Autodesk Fusion 360 part; units mm, degrees
(part 2 of 2)
sketch "Sketch5" plane through (0, 0, 0) normal (0, 1, 0) x (1, 0, 0)
  line L0 (-114.6631, -42.9541) -> (-114.6631, -45.4541)
  line L1 (-114.6631, -45.4541) -> (-84.6631, -45.4541)
  line L2 (-84.6631, -45.4541) -> (-84.6631, -42.9541)
  line L3 (-84.6631, -42.9541) -> (-114.6631, -42.9541)
  line L4 (-181.3297, -42.9541) -> (-181.3297, -45.4541)
  line L5 (-181.3297, -45.4541) -> (-151.3297, -45.4541)
  line L6 (-151.3297, -45.4541) -> (-151.3297, -42.9541)
  line L7 (-151.3297, -42.9541) -> (-181.3297, -42.9541)
  line L8 (-247.9964, -42.9541) -> (-247.9964, -45.4541)
  line L9 (-247.9964, -45.4541) -> (-217.9964, -45.4541)
  line L10 (-217.9964, -45.4541) -> (-217.9964, -42.9541)
  line L11 (-217.9964, -42.9541) -> (-247.9964, -42.9541)
  line L12 (-314.6631, -42.9541) -> (-314.6631, -45.4541)
  line L13 (-314.6631, -45.4541) -> (-284.6631, -45.4541)
  line L14 (-284.6631, -45.4541) -> (-284.6631, -42.9541)
  line L15 (-284.6631, -42.9541) -> (-314.6631, -42.9541)
  line L16 (-181.3297, -80.9541) -> (-181.3297, -83.4541)
  line L17 (-181.3297, -83.4541) -> (-151.3297, -83.4541)
  line L18 (-151.3297, -83.4541) -> (-151.3297, -80.9541)
  line L19 (-151.3297, -80.9541) -> (-181.3297, -80.9541)
  line L20 (-114.6631, -80.9541) -> (-114.6631, -83.4541)
  line L21 (-114.6631, -83.4541) -> (-84.6631, -83.4541)
  line L22 (-84.6631, -83.4541) -> (-84.6631, -80.9541)
  line L23 (-84.6631, -80.9541) -> (-114.6631, -80.9541)
  line L24 (-314.6631, -156.9541) -> (-314.6631, -159.4541)
  line L25 (-314.6631, -159.4541) -> (-284.6631, -159.4541)
  line L26 (-284.6631, -159.4541) -> (-284.6631, -156.9541)
  line L27 (-284.6631, -156.9541) -> (-314.6631, -156.9541)
  line L28 (-114.6631, -194.9541) -> (-114.6631, -197.4541)
  line L29 (-114.6631, -197.4541) -> (-84.6631, -197.4541)
  line L30 (-84.6631, -197.4541) -> (-84.6631, -194.9541)
  line L31 (-84.6631, -194.9541) -> (-114.6631, -194.9541)
  line L32 (-181.3297, -194.9541) -> (-181.3297, -197.4541)
  line L33 (-181.3297, -197.4541) -> (-151.3297, -197.4541)
  line L34 (-151.3297, -197.4541) -> (-151.3297, -194.9541)
  line L35 (-151.3297, -194.9541) -> (-181.3297, -194.9541)
  line L36 (-247.9964, -194.9541) -> (-247.9964, -197.4541)
  line L37 (-247.9964, -197.4541) -> (-217.9964, -197.4541)
  line L38 (-217.9964, -197.4541) -> (-217.9964, -194.9541)
  line L39 (-217.9964, -194.9541) -> (-247.9964, -194.9541)
  line L40 (-314.6631, -194.9541) -> (-314.6631, -197.4541)
  line L41 (-314.6631, -197.4541) -> (-284.6631, -197.4541)
  line L42 (-284.6631, -197.4541) -> (-284.6631, -194.9541)
  line L43 (-284.6631, -194.9541) -> (-314.6631, -194.9541)
  line L44 (-114.6631, -232.9541) -> (-114.6631, -235.4541)
  line L45 (-114.6631, -235.4541) -> (-84.6631, -235.4541)
  line L46 (-84.6631, -235.4541) -> (-84.6631, -232.9541)
  line L47 (-84.6631, -232.9541) -> (-114.6631, -232.9541)
  line L48 (-181.3297, -232.9541) -> (-181.3297, -235.4541)
  line L49 (-181.3297, -235.4541) -> (-151.3297, -235.4541)
  line L50 (-151.3297, -235.4541) -> (-151.3297, -232.9541)
  line L51 (-151.3297, -232.9541) -> (-181.3297, -232.9541)
  line L52 (-247.9964, -232.9541) -> (-247.9964, -235.4541)
  line L53 (-247.9964, -235.4541) -> (-217.9964, -235.4541)
  line L54 (-217.9964, -235.4541) -> (-217.9964, -232.9541)
  line L55 (-217.9964, -232.9541) -> (-247.9964, -232.9541)
  line L56 (-314.6631, -232.9541) -> (-314.6631, -235.4541)
  line L57 (-314.6631, -235.4541) -> (-284.6631, -235.4541)
  line L58 (-284.6631, -235.4541) -> (-284.6631, -232.9541)
  line L59 (-284.6631, -232.9541) -> (-314.6631, -232.9541)
  line L60 (-314.6631, -80.9541) -> (-314.6631, -83.4541)
  line L61 (-314.6631, -83.4541) -> (-284.6631, -83.4541)
  line L62 (-284.6631, -83.4541) -> (-284.6631, -80.9541)
  line L63 (-284.6631, -80.9541) -> (-314.6631, -80.9541)
  line L64 (-247.9964, -118.9541) -> (-247.9964, -121.4541)
  line L65 (-247.9964, -121.4541) -> (-217.9964, -121.4541)
  line L66 (-217.9964, -121.4541) -> (-217.9964, -118.9541)
  line L67 (-217.9964, -118.9541) -> (-247.9964, -118.9541)
  line L68 (-247.9964, -80.9541) -> (-247.9964, -83.4541)
  line L69 (-247.9964, -83.4541) -> (-217.9964, -83.4541)
  line L70 (-217.9964, -83.4541) -> (-217.9964, -80.9541)
  line L71 (-217.9964, -80.9541) -> (-247.9964, -80.9541)
  line L72 (-181.3297, -118.9541) -> (-181.3297, -121.4541)
  line L73 (-181.3297, -121.4541) -> (-151.3297, -121.4541)
  line L74 (-151.3297, -121.4541) -> (-151.3297, -118.9541)
  line L75 (-151.3297, -118.9541) -> (-181.3297, -118.9541)
  line L76 (-114.6631, -118.9541) -> (-114.6631, -121.4541)
  line L77 (-114.6631, -121.4541) -> (-84.6631, -121.4541)
  line L78 (-84.6631, -121.4541) -> (-84.6631, -118.9541)
  line L79 (-84.6631, -118.9541) -> (-114.6631, -118.9541)
  line L80 (-247.9964, -156.9541) -> (-247.9964, -159.4541)
  line L81 (-247.9964, -159.4541) -> (-217.9964, -159.4541)
  line L82 (-217.9964, -159.4541) -> (-217.9964, -156.9541)
  line L83 (-217.9964, -156.9541) -> (-247.9964, -156.9541)
  line L84 (-181.3297, -156.9541) -> (-181.3297, -159.4541)
  line L85 (-181.3297, -159.4541) -> (-151.3297, -159.4541)
  line L86 (-151.3297, -159.4541) -> (-151.3297, -156.9541)
  line L87 (-151.3297, -156.9541) -> (-181.3297, -156.9541)
  line L88 (-114.6631, -156.9541) -> (-114.6631, -159.4541)
  line L89 (-114.6631, -159.4541) -> (-84.6631, -159.4541)
  line L90 (-84.6631, -159.4541) -> (-84.6631, -156.9541)
  line L91 (-84.6631, -156.9541) -> (-114.6631, -156.9541)
  line L92 (-314.6631, -118.9541) -> (-314.6631, -121.4541)
  line L93 (-314.6631, -121.4541) -> (-284.6631, -121.4541)
  line L94 (-284.6631, -121.4541) -> (-284.6631, -118.9541)
  line L95 (-284.6631, -118.9541) -> (-314.6631, -118.9541)
  line L96 (-347.5, -182.5558) -> (-350, -182.5558)
  line L97 (-350, -182.5558) -> (-350, -154.875)
  line L98 (-350, -154.875) -> (-347.5, -154.875)
  line L99 (-347.5, -154.875) -> (-347.5, -115.125)
  line L100 (-347.5, -115.125) -> (-350, -115.125)
  line L101 (-350, -115.125) -> (-350, -87.4442)
  line L102 (-350, -87.4442) -> (-347.5, -87.4442)
  line L103 (-347.5, -87.4442) -> (-347.5, -47.6942)
  line L104 (-347.5, -47.6942) -> (-350, -47.6942)
  line L105 (-350, -47.6942) -> (-350, -10)
  line L106 (-350, -10) -> (-316.8881, -10)
  line L107 (-316.8881, -10) -> (-316.8881, -12.5)
  line L108 (-316.8881, -12.5) -> (-277.1381, -12.5)
  line L109 (-277.1381, -12.5) -> (-277.1381, -10)
  line L110 (-277.1381, -10) -> (-219.9429, -10)
  line L111 (-219.9429, -10) -> (-219.9429, -12.5)
  line L112 (-219.9429, -12.5) -> (-180.1929, -12.5)
  line L113 (-180.1929, -12.5) -> (-180.1929, -10)
  line L114 (-180.1929, -10) -> (-122.8387, -10)
  line L115 (-122.8387, -10) -> (-122.8387, -12.5)
  line L116 (-122.8387, -12.5) -> (-83.0887, -12.5)
  line L117 (-83.0887, -12.5) -> (-83.0887, -10)
  line L118 (-83.0887, -10) -> (-50, -10)
  line L119 (-50, -10) -> (-50, -47.6942)
  line L120 (-50, -47.6942) -> (-52.5, -47.6942)
  line L121 (-52.5, -47.6942) -> (-52.5, -87.4442)
  line L122 (-52.5, -87.4442) -> (-50, -87.4442)
  line L123 (-50, -87.4442) -> (-50, -115.125)
  line L124 (-50, -115.125) -> (-52.5, -115.125)
  line L125 (-52.5, -115.125) -> (-52.5, -154.875)
  line L126 (-52.5, -154.875) -> (-50, -154.875)
  line L127 (-50, -154.875) -> (-50, -182.5558)
  line L128 (-50, -182.5558) -> (-52.5, -182.5558)
  line L129 (-52.5, -182.5558) -> (-52.5, -222.3058)
  line L130 (-52.5, -222.3058) -> (-50, -222.3058)
  line L131 (-50, -222.3058) -> (-50, -260)
  line L132 (-50, -260) -> (-350, -260)
  line L133 (-350, -260) -> (-350, -222.3058)
  line L134 (-350, -222.3058) -> (-347.5, -222.3058)
  line L135 (-347.5, -222.3058) -> (-347.5, -182.5558)
  line L136 (-350, -382.5617) -> (-350, -362.5617)
  line L137 (-350, -362.5617) -> (-314.6631, -362.5617)
  line L138 (-314.6631, -362.5617) -> (-314.6631, -282.5617)
  line L139 (-314.6631, -282.5617) -> (-284.6631, -282.5617)
  line L140 (-284.6631, -282.5617) -> (-284.6631, -362.5617)
  line L141 (-284.6631, -362.5617) -> (-247.9964, -362.5617)
  line L142 (-247.9964, -362.5617) -> (-247.9964, -282.5617)
  line L143 (-247.9964, -282.5617) -> (-217.9964, -282.5617)
  line L144 (-217.9964, -282.5617) -> (-217.9964, -362.5617)
  line L145 (-217.9964, -362.5617) -> (-181.3297, -362.5617)
  line L146 (-181.3297, -362.5617) -> (-181.3297, -282.5617)
  line L147 (-181.3297, -282.5617) -> (-151.3297, -282.5617)
  line L148 (-151.3297, -282.5617) -> (-151.3297, -362.5617)
  line L149 (-151.3297, -362.5617) -> (-114.6631, -362.5617)
  line L150 (-114.6631, -362.5617) -> (-114.6631, -282.5617)
  line L151 (-114.6631, -282.5617) -> (-84.6631, -282.5617)
  line L152 (-84.6631, -282.5617) -> (-84.6631, -362.5617)
  line L153 (-84.6631, -362.5617) -> (-50, -362.5617)
  line L154 (-50, -362.5617) -> (-50, -382.5617)
  arc A0 (-60, -392.5617) -> (-50, -382.5617) centre (-60, -382.5617) ccw
  line L155 (-60, -392.5617) -> (-340, -392.5617)
  arc A1 (-350, -382.5617) -> (-340, -392.5617) centre (-340, -382.5617) ccw
  line L156 (0, -357.5617) -> (0, -337.5617)
  line L157 (0, -337.5617) -> (35.3369, -337.5617)
  line L158 (35.3369, -337.5617) -> (35.3369, -257.5617)
  line L159 (35.3369, -257.5617) -> (65.3369, -257.5617)
  line L160 (65.3369, -257.5617) -> (65.3369, -337.5617)
  line L161 (65.3369, -337.5617) -> (102.0036, -337.5617)
  line L162 (102.0036, -337.5617) -> (102.0036, -257.5617)
  line L163 (102.0036, -257.5617) -> (132.0036, -257.5617)
  line L164 (132.0036, -257.5617) -> (132.0036, -337.5617)
  line L165 (132.0036, -337.5617) -> (168.6703, -337.5617)
  line L166 (168.6703, -337.5617) -> (168.6703, -257.5617)
  line L167 (168.6703, -257.5617) -> (198.6703, -257.5617)
  line L168 (198.6703, -257.5617) -> (198.6703, -337.5617)
  line L169 (198.6703, -337.5617) -> (235.3369, -337.5617)
  line L170 (235.3369, -337.5617) -> (235.3369, -257.5617)
  line L171 (235.3369, -257.5617) -> (265.3369, -257.5617)
  line L172 (265.3369, -257.5617) -> (265.3369, -337.5617)
  line L173 (265.3369, -337.5617) -> (300, -337.5617)
  line L174 (300, -337.5617) -> (300, -357.5617)
  arc A2 (290, -367.5617) -> (300, -357.5617) centre (290, -357.5617) ccw
  line L175 (290, -367.5617) -> (10, -367.5617)
  arc A3 (0, -357.5617) -> (10, -367.5617) centre (10, -357.5617) ccw
  line L176 (235.3369, -32.9541) -> (235.3369, -35.4541)
  line L177 (235.3369, -35.4541) -> (265.3369, -35.4541)
  line L178 (265.3369, -35.4541) -> (265.3369, -32.9541)
  line L179 (265.3369, -32.9541) -> (235.3369, -32.9541)
  line L180 (168.6703, -32.9541) -> (168.6703, -35.4541)
  line L181 (168.6703, -35.4541) -> (198.6703, -35.4541)
  line L182 (198.6703, -35.4541) -> (198.6703, -32.9541)
  line L183 (198.6703, -32.9541) -> (168.6703, -32.9541)
  line L184 (102.0036, -32.9541) -> (102.0036, -35.4541)
  line L185 (102.0036, -35.4541) -> (132.0036, -35.4541)
  line L186 (132.0036, -35.4541) -> (132.0036, -32.9541)
  line L187 (132.0036, -32.9541) -> (102.0036, -32.9541)
  line L188 (35.3369, -32.9541) -> (35.3369, -35.4541)
  line L189 (35.3369, -35.4541) -> (65.3369, -35.4541)
  line L190 (65.3369, -35.4541) -> (65.3369, -32.9541)
  line L191 (65.3369, -32.9541) -> (35.3369, -32.9541)
  line L192 (168.6703, -70.9541) -> (168.6703, -73.4541)
  line L193 (168.6703, -73.4541) -> (198.6703, -73.4541)
  line L194 (198.6703, -73.4541) -> (198.6703, -70.9541)
  line L195 (198.6703, -70.9541) -> (168.6703, -70.9541)
  line L196 (235.3369, -70.9541) -> (235.3369, -73.4541)
  line L197 (235.3369, -73.4541) -> (265.3369, -73.4541)
  line L198 (265.3369, -73.4541) -> (265.3369, -70.9541)
  line L199 (265.3369, -70.9541) -> (235.3369, -70.9541)
  line L200 (35.3369, -146.9541) -> (35.3369, -149.4541)
  line L201 (35.3369, -149.4541) -> (65.3369, -149.4541)
  line L202 (65.3369, -149.4541) -> (65.3369, -146.9541)
  line L203 (65.3369, -146.9541) -> (35.3369, -146.9541)
  line L204 (235.3369, -184.9541) -> (235.3369, -187.4541)
  line L205 (235.3369, -187.4541) -> (265.3369, -187.4541)
  line L206 (265.3369, -187.4541) -> (265.3369, -184.9541)
  line L207 (265.3369, -184.9541) -> (235.3369, -184.9541)
  line L208 (168.6703, -184.9541) -> (168.6703, -187.4541)
  line L209 (168.6703, -187.4541) -> (198.6703, -187.4541)
  line L210 (198.6703, -187.4541) -> (198.6703, -184.9541)
  line L211 (198.6703, -184.9541) -> (168.6703, -184.9541)
  line L212 (102.0036, -184.9541) -> (102.0036, -187.4541)
  line L213 (102.0036, -187.4541) -> (132.0036, -187.4541)
  line L214 (132.0036, -187.4541) -> (132.0036, -184.9541)
  line L215 (132.0036, -184.9541) -> (102.0036, -184.9541)
  line L216 (35.3369, -184.9541) -> (35.3369, -187.4541)
  line L217 (35.3369, -187.4541) -> (65.3369, -187.4541)
  line L218 (65.3369, -187.4541) -> (65.3369, -184.9541)
  line L219 (65.3369, -184.9541) -> (35.3369, -184.9541)
  line L220 (235.3369, -222.9541) -> (235.3369, -225.4541)
  line L221 (235.3369, -225.4541) -> (265.3369, -225.4541)
  line L222 (265.3369, -225.4541) -> (265.3369, -222.9541)
  line L223 (265.3369, -222.9541) -> (235.3369, -222.9541)
  line L224 (168.6703, -222.9541) -> (168.6703, -225.4541)
  line L225 (168.6703, -225.4541) -> (198.6703, -225.4541)
  line L226 (198.6703, -225.4541) -> (198.6703, -222.9541)
  line L227 (198.6703, -222.9541) -> (168.6703, -222.9541)
  line L228 (102.0036, -222.9541) -> (102.0036, -225.4541)
  line L229 (102.0036, -225.4541) -> (132.0036, -225.4541)
  line L230 (132.0036, -225.4541) -> (132.0036, -222.9541)
  line L231 (132.0036, -222.9541) -> (102.0036, -222.9541)
  line L232 (35.3369, -222.9541) -> (35.3369, -225.4541)
  line L233 (35.3369, -225.4541) -> (65.3369, -225.4541)
  line L234 (65.3369, -225.4541) -> (65.3369, -222.9541)
  line L235 (65.3369, -222.9541) -> (35.3369, -222.9541)
  line L236 (35.3369, -70.9541) -> (35.3369, -73.4541)
  line L237 (35.3369, -73.4541) -> (65.3369, -73.4541)
  line L238 (65.3369, -73.4541) -> (65.3369, -70.9541)
  line L239 (65.3369, -70.9541) -> (35.3369, -70.9541)
  line L240 (102.0036, -108.9541) -> (102.0036, -111.4541)
  line L241 (102.0036, -111.4541) -> (132.0036, -111.4541)
  line L242 (132.0036, -111.4541) -> (132.0036, -108.9541)
  line L243 (132.0036, -108.9541) -> (102.0036, -108.9541)
  line L244 (102.0036, -70.9541) -> (102.0036, -73.4541)
  line L245 (102.0036, -73.4541) -> (132.0036, -73.4541)
  line L246 (132.0036, -73.4541) -> (132.0036, -70.9541)
  line L247 (132.0036, -70.9541) -> (102.0036, -70.9541)
  line L248 (168.6703, -108.9541) -> (168.6703, -111.4541)
  line L249 (168.6703, -111.4541) -> (198.6703, -111.4541)
  line L250 (198.6703, -111.4541) -> (198.6703, -108.9541)
  line L251 (198.6703, -108.9541) -> (168.6703, -108.9541)
  line L252 (235.3369, -108.9541) -> (235.3369, -111.4541)
  line L253 (235.3369, -111.4541) -> (265.3369, -111.4541)
  line L254 (265.3369, -111.4541) -> (265.3369, -108.9541)
  line L255 (265.3369, -108.9541) -> (235.3369, -108.9541)
  line L256 (102.0036, -146.9541) -> (102.0036, -149.4541)
  line L257 (102.0036, -149.4541) -> (132.0036, -149.4541)
  line L258 (132.0036, -149.4541) -> (132.0036, -146.9541)
  line L259 (132.0036, -146.9541) -> (102.0036, -146.9541)
  line L260 (168.6703, -146.9541) -> (168.6703, -149.4541)
  line L261 (168.6703, -149.4541) -> (198.6703, -149.4541)
  line L262 (198.6703, -149.4541) -> (198.6703, -146.9541)
  line L263 (198.6703, -146.9541) -> (168.6703, -146.9541)
  line L264 (235.3369, -146.9541) -> (235.3369, -149.4541)
  line L265 (235.3369, -149.4541) -> (265.3369, -149.4541)
  line L266 (265.3369, -149.4541) -> (265.3369, -146.9541)
  line L267 (265.3369, -146.9541) -> (235.3369, -146.9541)
  line L268 (35.3369, -108.9541) -> (35.3369, -111.4541)
  line L269 (35.3369, -111.4541) -> (65.3369, -111.4541)
  line L270 (65.3369, -111.4541) -> (65.3369, -108.9541)
  line L271 (65.3369, -108.9541) -> (35.3369, -108.9541)
  line L272 (2.5, -172.5558) -> (0, -172.5558)
  line L273 (0, -172.5558) -> (0, -144.875)
  line L274 (0, -144.875) -> (2.5, -144.875)
  line L275 (2.5, -144.875) -> (2.5, -105.125)
  line L276 (2.5, -105.125) -> (0, -105.125)
  line L277 (0, -105.125) -> (0, -77.4442)
  line L278 (0, -77.4442) -> (2.5, -77.4442)
  line L279 (2.5, -77.4442) -> (2.5, -37.6942)
  line L280 (2.5, -37.6942) -> (0, -37.6942)
  line L281 (0, -37.6942) -> (0, 0)
  line L282 (0, 0) -> (33.1119, 0)
  line L283 (33.1119, 0) -> (33.1119, -2.5)
  line L284 (33.1119, -2.5) -> (72.8619, -2.5)
  line L285 (72.8619, -2.5) -> (72.8619, 0)
  line L286 (72.8619, 0) -> (130.0571, 0)
  line L287 (130.0571, 0) -> (130.0571, -2.5)
  line L288 (130.0571, -2.5) -> (169.8071, -2.5)
  line L289 (169.8071, -2.5) -> (169.8071, 0)
  line L290 (169.8071, 0) -> (227.1613, 0)
  line L291 (227.1613, 0) -> (227.1613, -2.5)
  line L292 (227.1613, -2.5) -> (266.9113, -2.5)
  line L293 (266.9113, -2.5) -> (266.9113, 0)
  line L294 (266.9113, 0) -> (300, 0)
  line L295 (300, 0) -> (300, -37.6942)
  line L296 (300, -37.6942) -> (297.5, -37.6942)
  line L297 (297.5, -37.6942) -> (297.5, -77.4442)
  line L298 (297.5, -77.4442) -> (300, -77.4442)
  line L299 (300, -77.4442) -> (300, -105.125)
  line L300 (300, -105.125) -> (297.5, -105.125)
  line L301 (297.5, -105.125) -> (297.5, -144.875)
  line L302 (297.5, -144.875) -> (300, -144.875)
  line L303 (300, -144.875) -> (300, -172.5558)
  line L304 (300, -172.5558) -> (297.5, -172.5558)
  line L305 (297.5, -172.5558) -> (297.5, -212.3058)
  line L306 (297.5, -212.3058) -> (300, -212.3058)
  line L307 (300, -212.3058) -> (300, -250)
  line L308 (300, -250) -> (0, -250)
  line L309 (0, -250) -> (0, -212.3058)
  line L310 (0, -212.3058) -> (2.5, -212.3058)
  line L311 (2.5, -212.3058) -> (2.5, -172.5558)
  line L312 (296.4708, 56.207) -> (296.4708, 12.1817)
  line L313 (296.4708, 12.1817) -> (265.8821, 12.1817)
  line L314 (265.8821, 12.1817) -> (265.8821, 9.6817)
  line L315 (265.8821, 9.6817) -> (225.8821, 9.6817)
  line L316 (225.8821, 9.6817) -> (225.8821, 12.1817)
  line L317 (225.8821, 12.1817) -> (168.5279, 12.1817)
  line L318 (168.5279, 12.1817) -> (168.5279, 9.6817)
  line L319 (168.5279, 9.6817) -> (129.2779, 9.6817)
  line L320 (129.2779, 9.6817) -> (129.2779, 12.1817)
  line L321 (129.2779, 12.1817) -> (72.0827, 12.1817)
  line L322 (72.0827, 12.1817) -> (72.0827, 9.6817)
  line L323 (72.0827, 9.6817) -> (32.0827, 9.6817)
  line L324 (32.0827, 9.6817) -> (32.0827, 12.1817)
  line L325 (32.0827, 12.1817) -> (1.4708, 12.1817)
  line L326 (1.4708, 12.1817) -> (1.4708, 56.207)
  line L327 (1.4708, 56.207) -> (-1.0292, 56.207)
  line L328 (-1.0292, 56.207) -> (-1.0292, 96.207)
  line L329 (-1.0292, 96.207) -> (1.4708, 96.207)
  line L330 (1.4708, 96.207) -> (1.4708, 139.6817)
  line L331 (1.4708, 139.6817) -> (-1.0292, 139.6817)
  line L332 (-1.0292, 139.6817) -> (-1.0292, 179.6817)
  line L333 (-1.0292, 179.6817) -> (1.4708, 179.6817)
  line L334 (1.4708, 179.6817) -> (1.4708, 223.1564)
  line L335 (1.4708, 223.1564) -> (-1.0292, 223.1564)
  line L336 (-1.0292, 223.1564) -> (-1.0292, 263.1564)
  line L337 (-1.0292, 263.1564) -> (1.4708, 263.1564)
  line L338 (1.4708, 263.1564) -> (1.4708, 307.1817)
  line L339 (1.4708, 307.1817) -> (32.0827, 307.1817)
  line L340 (32.0827, 307.1817) -> (32.0827, 309.6817)
  line L341 (32.0827, 309.6817) -> (72.0827, 309.6817)
  line L342 (72.0827, 309.6817) -> (72.0827, 307.1817)
  line L343 (72.0827, 307.1817) -> (129.2779, 307.1817)
  line L344 (129.2779, 307.1817) -> (129.2779, 309.6817)
  line L345 (129.2779, 309.6817) -> (168.5279, 309.6817)
  line L346 (168.5279, 309.6817) -> (168.5279, 307.1817)
  line L347 (168.5279, 307.1817) -> (225.8821, 307.1817)
  line L348 (225.8821, 307.1817) -> (225.8821, 309.6817)
  line L349 (225.8821, 309.6817) -> (265.8821, 309.6817)
  line L350 (265.8821, 309.6817) -> (265.8821, 307.1817)
  line L351 (265.8821, 307.1817) -> (296.4708, 307.1817)
  line L352 (296.4708, 307.1817) -> (296.4708, 263.1564)
  line L353 (296.4708, 263.1564) -> (298.9708, 263.1564)
  line L354 (298.9708, 263.1564) -> (298.9708, 223.1564)
  line L355 (298.9708, 223.1564) -> (296.4708, 223.1564)
  line L356 (296.4708, 223.1564) -> (296.4708, 179.6817)
  line L357 (296.4708, 179.6817) -> (298.9708, 179.6817)
  line L358 (298.9708, 179.6817) -> (298.9708, 139.6817)
  line L359 (298.9708, 139.6817) -> (296.4708, 139.6817)
  line L360 (296.4708, 139.6817) -> (296.4708, 96.207)
  line L361 (296.4708, 96.207) -> (298.9708, 96.207)
  line L362 (298.9708, 96.207) -> (298.9708, 56.207)
  line L363 (298.9708, 56.207) -> (296.4708, 56.207)
  line L364 (-18.915, 96.082) -> (-21.415, 96.082)
  line L365 (-21.415, 96.082) -> (-21.415, 56.332)
  line L366 (-21.415, 56.332) -> (-18.915, 56.332)
  line L367 (-18.915, 56.332) -> (-18.915, 12.1817)
  line L368 (-18.915, 12.1817) -> (-56.6092, 12.1817)
  line L369 (-56.6092, 12.1817) -> (-56.6092, 9.6817)
  line L370 (-56.6092, 9.6817) -> (-96.6092, 9.6817)
  line L371 (-96.6092, 9.6817) -> (-96.6092, 12.1817)
  line L372 (-96.6092, 12.1817) -> (-123.54, 12.1817)
  line L373 (-123.54, 12.1817) -> (-123.54, 9.6817)
  line L374 (-123.54, 9.6817) -> (-163.54, 9.6817)
  line L375 (-163.54, 9.6817) -> (-163.54, 12.1817)
  line L376 (-163.54, 12.1817) -> (-191.2208, 12.1817)
  line L377 (-191.2208, 12.1817) -> (-191.2208, 9.6817)
  line L378 (-191.2208, 9.6817) -> (-231.2208, 9.6817)
  line L379 (-231.2208, 9.6817) -> (-231.2208, 12.1817)
  line L380 (-231.2208, 12.1817) -> (-268.915, 12.1817)
  line L381 (-268.915, 12.1817) -> (-268.915, 307.1817)
  line L382 (-268.915, 307.1817) -> (-231.2208, 307.1817)
  line L383 (-231.2208, 307.1817) -> (-231.2208, 309.6817)
  line L384 (-231.2208, 309.6817) -> (-191.2208, 309.6817)
  line L385 (-191.2208, 309.6817) -> (-191.2208, 307.1817)
  line L386 (-191.2208, 307.1817) -> (-163.54, 307.1817)
  line L387 (-163.54, 307.1817) -> (-163.54, 309.6817)
  line L388 (-163.54, 309.6817) -> (-123.54, 309.6817)
  line L389 (-123.54, 309.6817) -> (-123.54, 307.1817)
  line L390 (-123.54, 307.1817) -> (-96.6092, 307.1817)
  line L391 (-96.6092, 307.1817) -> (-96.6092, 309.6817)
  line L392 (-96.6092, 309.6817) -> (-56.6092, 309.6817)
  line L393 (-56.6092, 309.6817) -> (-56.6092, 307.1817)
  line L394 (-56.6092, 307.1817) -> (-18.915, 307.1817)
  line L395 (-18.915, 307.1817) -> (-18.915, 263.0314)
  line L396 (-18.915, 263.0314) -> (-21.415, 263.0314)
  line L397 (-21.415, 263.0314) -> (-21.415, 223.2814)
  line L398 (-21.415, 223.2814) -> (-18.915, 223.2814)
  line L399 (-18.915, 223.2814) -> (-18.915, 179.4138)
  line L400 (-18.915, 179.4138) -> (-21.415, 179.4138)
  line L401 (-21.415, 179.4138) -> (-21.415, 139.6638)
  line L402 (-21.415, 139.6638) -> (-18.915, 139.6638)
  line L403 (-18.915, 139.6638) -> (-18.915, 96.082)
  line L404 (281.085, 446.082) -> (278.585, 446.082)
  line L405 (278.585, 446.082) -> (278.585, 406.332)
  line L406 (278.585, 406.332) -> (281.085, 406.332)
  line L407 (281.085, 406.332) -> (281.085, 362.1817)
  line L408 (281.085, 362.1817) -> (243.3908, 362.1817)
  line L409 (243.3908, 362.1817) -> (243.3908, 359.6817)
  line L410 (243.3908, 359.6817) -> (203.3908, 359.6817)
  line L411 (203.3908, 359.6817) -> (203.3908, 362.1817)
  line L412 (203.3908, 362.1817) -> (176.46, 362.1817)
  line L413 (176.46, 362.1817) -> (176.46, 359.6817)
  line L414 (176.46, 359.6817) -> (136.46, 359.6817)
  line L415 (136.46, 359.6817) -> (136.46, 362.1817)
  line L416 (136.46, 362.1817) -> (108.7792, 362.1817)
  line L417 (108.7792, 362.1817) -> (108.7792, 359.6817)
  line L418 (108.7792, 359.6817) -> (68.7792, 359.6817)
  line L419 (68.7792, 359.6817) -> (68.7792, 362.1817)
  line L420 (68.7792, 362.1817) -> (31.085, 362.1817)
  line L421 (31.085, 362.1817) -> (31.085, 657.1817)
  line L422 (31.085, 657.1817) -> (68.7792, 657.1817)
  line L423 (68.7792, 657.1817) -> (68.7792, 659.6817)
  line L424 (68.7792, 659.6817) -> (108.7792, 659.6817)
  line L425 (108.7792, 659.6817) -> (108.7792, 657.1817)
  line L426 (108.7792, 657.1817) -> (136.46, 657.1817)
  line L427 (136.46, 657.1817) -> (136.46, 659.6817)
  line L428 (136.46, 659.6817) -> (176.46, 659.6817)
  line L429 (176.46, 659.6817) -> (176.46, 657.1817)
  line L430 (176.46, 657.1817) -> (203.3908, 657.1817)
  line L431 (203.3908, 657.1817) -> (203.3908, 659.6817)
  line L432 (203.3908, 659.6817) -> (243.3908, 659.6817)
  line L433 (243.3908, 659.6817) -> (243.3908, 657.1817)
  line L434 (243.3908, 657.1817) -> (281.085, 657.1817)
  line L435 (281.085, 657.1817) -> (281.085, 613.0314)
  line L436 (281.085, 613.0314) -> (278.585, 613.0314)
  line L437 (278.585, 613.0314) -> (278.585, 573.2814)
  line L438 (278.585, 573.2814) -> (281.085, 573.2814)
  line L439 (281.085, 573.2814) -> (281.085, 529.4138)
  line L440 (281.085, 529.4138) -> (278.585, 529.4138)
  line L441 (278.585, 529.4138) -> (278.585, 489.6638)
  line L442 (278.585, 489.6638) -> (281.085, 489.6638)
  line L443 (281.085, 489.6638) -> (281.085, 446.082)
component "front" placed x (1, 0, 0) y (0, 1, 0) z (0, 0, 1) at (0, 0, 0)
component "side" placed x (1, 0, 0) y (0, 1, 0) z (0, 0, 1) at (0, 0, 0)
component "base" placed x (1, 0, 0) y (0, 1, 0) z (0, 0, 1) at (0, 0, 0)
component "frontbis" placed x (1, 0, 0) y (0, 1, 0) z (0, 0, 1) at (0, 0, 0)
component "sidebis" placed x (1, 0, 0) y (0, 1, 0) z (0, 0, 1) at (0, 0, 0)
component "ruler" placed x (1, 0, 0) y (0, 1, 0) z (0, 0, 1) at (0, 0, 0)
component "ruler2" placed x (1, 0, 0) y (0, 1, 0) z (0, 0, 1) at (0, 0, 0)
component "front" placed x (1, 0, 0) y (0, 1, 0) z (0, 0, 1) at (-350, 0, 10) in component "frontbis"
component "side" placed x (1, 0, 0) y (0, 1, 0) z (0, 0, 1) at (300, 0, -350) in component "sidebis"
component "ruler" placed x (1, 0, 0) y (0, 1, 0) z (0, 0, 1) at (-350, 0, 25) in component "ruler2"
equation "length = 300 mm"
equation "height = 250 mm"
equation "d3 = length"
equation "d4 = height"
equation "thickness = 2.5 mm"
equation "width = 300 mm"
equation "d14 = tooth - kerf"
equation "d15 = tooth - kerf"
equation "tooth = 40 mm"
equation "d17 = tooth - kerf"
equation "d18 = tooth - kerf"
equation "d19 = thickness"
equation "d20 = tooth - kerf"
equation "d21 = thickness"
equation "d22 = tooth - kerf"
equation "d23 = thickness"
equation "d24 = tooth - kerf"
equation "d25 = tooth - kerf"
equation "d26 = tooth - kerf"
equation "d27 = thickness"
equation "d28 = thickness"
equation "d29 = thickness"
equation "d31 = height"
equation "d32 = width"
equation "d33 = thickness"
equation "d36 = thickness"
equation "d37 = tooth"
equation "d38 = thickness"
equation "d39 = thickness"
equation "d40 = tooth"
equation "d41 = tooth"
equation "d45 = length"
equation "d46 = width"
equation "d47 = thickness"
equation "d48 = thickness"
equation "d49 = tooth"
equation "d50 = thickness"
equation "d51 = thickness"
equation "d52 = tooth"
equation "d54 = thickness"
equation "d55 = thickness"
equation "d56 = tooth"
equation "d58 = thickness"
equation "d60 = thickness"
equation "d61 = tooth"
equation "d62 = tooth"
equation "d64 = thickness"
equation "d66 = tooth - kerf"
equation "d67 = thickness"
equation "d69 = tooth - kerf"
equation "d70 = thickness"
equation "d71 = thickness"
equation "d72 = tooth - kerf"
equation "kerf = 0.25 mm"
equation "d81 = thickness"
equation "ruler_finger = 30 mm"
equation "d85 = ruler_finger"
equation "d86 = thickness"
equation "d91 = length"
equation "d98 = ruler_finger"
equation "d99 = ruler_finger"
equation "d100 = ruler_finger"
equation "d101 = ruler_finger"
equation "d102 = thickness"
